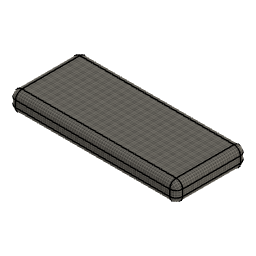
bed structure (Autodesk Fusion 360 archive; units mm, degrees)
design "mattress"
Autodesk Fusion 360 part; units mm, degrees
sketch "Sketch1" plane through (0, 0, 0) normal (0, 0, 1) x (1, 0, 0)
  line L0 (0, 50) -> (130, 50)
  line L1 (130, 50) -> (130, -5)
  line L2 (130, -5) -> (0, -5)
  line L3 (0, -5) -> (0, 50)
  dimension "d1" = 55
  dimension "d2" = 130
  constraint horizontal L0
  constraint vertical L1
  constraint horizontal L2
  constraint vertical L3
  measures "d1" distance of L0.start L2.end
  measures "d2" distance of L0.start L0.end
extrude "Extrude1" add sketch "Sketch1" along normal blind 15
fillet "Fillet1" radius 5 4 faces at (130, 31.6667, 5) (86.6667, -5, 5) (43.3333, 50, 5) (0, 13.3333, 5)
